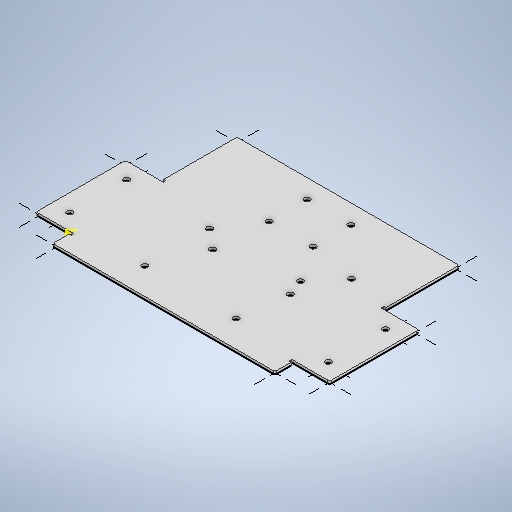
# Autodesk Inventor part: body_middle_frame
Saved by Autodesk Inventor 2026.1 (Build 301233000, 233)
## iProperties
Created: 2025-08-16
Part Number: body_middle_frame
Material: Generic
Document SubType Name: Modeling
Designer: chris
Density: 1 g/cm^3
Appearance: Default
Author: chris
Autodesk Inventor part; units mm, degrees
ref_plane "YZ Plane" through (0, 0, 0) normal (1, 0, 0) x (0, 1, 0)
ref_plane "XZ Plane" through (0, 0, 0) normal (0, 1, 0) x (-1, 0, 0)
ref_plane "XY Plane" through (0, 0, 0) normal (0, 0, 1) x (1, 0, 0)
sketch "Sketch2" plane through (0, 0, 0) normal (0, 1, 0) x (-1, 0, 0)
  line L0 (-0.4496, -47) -> (-0.4496, 0)
  line L1 (-117.7289, 0) -> (-117.7289, -47)
  circle A0 centre (-86.4344, -29.299) radius 1.55
  circle A1 centre (-45.3894, -29.3) radius 1.55
  circle A2 centre (-95.4122, -52.4581) radius 1.55
  circle A3 centre (-83.0893, -4) radius 1.55
  circle A4 centre (-35.0893, -4) radius 1.55
  circle A5 centre (-83.0893, -38) radius 1.55
  circle A6 centre (-35.0893, -38) radius 1.55
  circle A7 centre (-70.6843, -57) radius 1.55
  circle A8 centre (-70.6843, -77) radius 1.55
  circle A9 centre (-47.4943, -57) radius 1.55
  circle A10 centre (-47.4943, -77) radius 1.55
  circle A11 centre (9.095, -8.5) radius 1.55
  circle A12 centre (-127.2736, -8.5) radius 1.55
  circle A13 centre (9.095, -38.5) radius 1.55
  circle A14 centre (-127.2736, -38.5) radius 1.55
  arc A15 (-117.5893, -86) -> (-116.5893, -87) centre (-116.5893, -86) ccw
  line L2 (-117.5893, -86) -> (-117.5893, -48.5)
  arc A16 (-136.3686, -46) -> (-135.3686, -47) centre (-135.3686, -46) ccw
  arc A17 (-135.3686, 0) -> (-136.3686, -1) centre (-135.3686, -1) ccw
  line L3 (-135.3686, 0) -> (-116.5293, 0)
  arc A18 (-116.5893, 10) -> (-117.5893, 9) centre (-116.5893, 9) ccw
  line L4 (-117.5893, 1.5) -> (-117.5893, 9)
  arc A19 (-0.5893, 9) -> (-1.5893, 10) centre (-1.5893, 9) ccw
  line L5 (-0.5893, 9) -> (-0.5893, 1.5)
  arc A20 (18.19, -1) -> (17.19, 0) centre (17.19, -1) ccw
  arc A21 (17.19, -47) -> (18.19, -46) centre (17.19, -46) ccw
  line L6 (17.19, -47) -> (-1.6493, -47)
  arc A22 (-1.5893, -87) -> (-0.5893, -86) centre (-1.5893, -86) ccw
  line L7 (-0.5893, -48.5) -> (-0.5893, -86)
  line L8 (-136.3686, -46) -> (-136.3686, -1)
  line L9 (18.19, -1) -> (18.19, -46)
  line L10 (-1.6493, 0) -> (17.19, 0)
  line L11 (-1.6493, 0) -> (-1.6493, 1.5)
  line L12 (-1.6493, 1.5) -> (-0.5893, 1.5)
  line L13 (-116.5893, 10) -> (-1.5893, 10)
  line L14 (-117.5893, 1.5) -> (-116.5293, 1.5)
  line L15 (-116.5293, 1.5) -> (-116.5293, 0)
  line L16 (-116.5293, -47) -> (-135.3686, -47)
  line L17 (-116.5293, -47) -> (-116.5293, -48.5)
  line L18 (-116.5293, -48.5) -> (-117.5893, -48.5)
  line L19 (-1.5893, -87) -> (-116.5893, -87)
  line L20 (-0.5893, -48.5) -> (-1.6493, -48.5)
  line L21 (-1.6493, -48.5) -> (-1.6493, -47)
  line L22 (-118.1786, -47) -> (-118.1786, 0)
  line L23 (-117.2793, 0) -> (-117.2793, -47)
  line L24 (-0.8993, -47) -> (-0.8993, 0)
  line L25 (0, 0) -> (0, -47)
  constraints: 52 end point, 23 centre point, 23 tangent, 21 equal radius, 16 parallel, 16 point on circle, 16 vertical, 12 point on line, 10 horizontal, 6 perpendicular, 87 other
extrude "Extrusion2" add sketch "Sketch2" along normal blind 1.5
body "Solid2"
